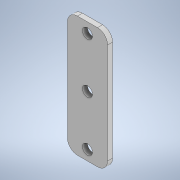
# Autodesk Inventor part: mitad
Saved by Autodesk Inventor 2022 (Build 260153000, 153)
## iProperties
Created: 2022-10-14
Part Number: mitad
Material: Generic
Document SubType Name: Modeling
Designer: Usuario
Density: 1 g/cm^3
Appearance: Default
Author: Usuario
Autodesk Inventor part; units mm, degrees
ref_plane "YZ Plane" through (0, 0, 0) normal (1, 0, 0) x (0, 1, 0)
ref_plane "XZ Plane" through (0, 0, 0) normal (0, 1, 0) x (-1, 0, 0)
ref_plane "XY Plane" through (0, 0, 0) normal (0, 0, 1) x (1, 0, 0)
sketch "Sketch1" plane through (0, 0, 0) normal (0, 0, 1) x (1, 0, 0)
  line L0 (-10, 60) -> (10, 60)
  line L1 (20, 50) -> (20, -50)
  line L2 (10, -60) -> (-10, -60)
  line L3 (-20, -50) -> (-20, 50)
  arc A0 (-10, 60) -> (-20, 50) centre (-10, 50) ccw
  arc A1 (20, 50) -> (10, 60) centre (10, 50) ccw
  arc A2 (10, -60) -> (20, -50) centre (10, -50) ccw
  arc A3 (-20, -50) -> (-10, -60) centre (-10, -50) ccw
  point P0 (0, 0)
  point P1 (20, 0)
  point P2 (0, 60)
  dimension "d0" = 10
  dimension "d1" = 40
  dimension "d2" = 120
  constraints: 8 end point, 8 point on circle, 8 tangent, 4 centre point, 3 equal radius, 2 midpoint, 2 parallel, 1 horizontal, 1 horizontal alignment, 1 perpendicular, 1 vertical alignment
  measures "d0" radius of A0
  measures "d1" distance between parallel lines of L1 L3
  measures "d2" distance between parallel lines of L2 L0
extrude "Extrusion1" add sketch "Sketch1" along normal blind 5
sketch "Sketch2" plane through (0, 0, 5) normal (0, 0, 1) x (1, 0, 0)
  circle A0 centre (0, 50) radius 5
  line L0 (-20, 50) -> (-20, -50) construction
  line L1 (-20, 0) -> (20, 0) construction
  line L2 (20, -50) -> (20, 50) construction
  line L3 (10, 60) -> (-10, 60) projected
  circle A1 centre (0, -50) radius 5
  circle A2 centre (0, 0) radius 5
  point P0 (0, 0)
  dimension "d5" = 10
  dimension "d7" = 10
  dimension "d8" = 10
  constraints: 3 centre point, 3 midpoint, 2 end point, 1 coincident, 1 symmetric about line, 1 vertical alignment, 1 other
  measures "d5" diameter of A0
  measures "d7" distance from line of L3 A0.centre
  measures "d8" diameter of A2
extrude "Extrusion2" cut sketch "Sketch2" against normal up to surface (5 mm away)
body "Solid1"
